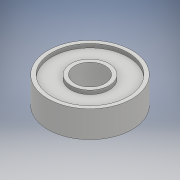
# Autodesk Inventor part: Подшипник
Saved by Autodesk Inventor 2017 (Build 210142000, 142)
## iProperties
Part Number: Подшипник
Material: Типовые
Document SubType Name: Modeling
Designer: Daemon
Density: 1 g/cm^3
Appearance: По умолчанию
Author: Daemon
Autodesk Inventor part; units mm, degrees
ref_plane "YZ Plane" through (0, 0, 0) normal (1, 0, 0) x (0, 1, 0)
ref_plane "XZ Plane" through (0, 0, 0) normal (0, 1, 0) x (-1, 0, 0)
ref_plane "XY Plane" through (0, 0, 0) normal (0, 0, 1) x (1, 0, 0)
sketch "Эскиз1" plane through (0, 0, 0) normal (0, 0, 1) x (1, 0, 0)
  circle A0 centre (0, 0) radius 4
  circle A1 centre (0, 0) radius 11
  dimension "d0" = 8
  dimension "d1" = 22
  constraints: 2 centre point, 2 coincident
  measures "d0" diameter of A0
  measures "d1" diameter of A1
extrude "Выдавливание1" add sketch "Эскиз1" along normal blind 7
sketch "Эскиз3" plane through (0, 0, 7) normal (0, 0, 1) x (1, 0, 0)
  circle A0 centre (0, 0) radius 4 projected
  circle A1 centre (0, 0) radius 4
  circle A2 centre (0, 0) radius 5
  circle A3 centre (0, 0) radius 10
  circle A4 centre (0, 0) radius 11
  dimension "d8" = 10
  dimension "d9" = 20
  dimension "d10" = 22
  dimension "d11" = 8
  constraints: 4 centre point, 4 coincident
  measures "d8" diameter of A2
  measures "d9" diameter of A3
  measures "d10" diameter of A4
  measures "d11" diameter of A1
extrude "Выдавливание3" cut sketch "Эскиз3" against normal blind 1 contours A3
sketch "Эскиз4" plane through (0, 0, 0) normal (0, 0, -1) x (-1, 0, 0)
  circle A0 centre (0, 0) radius 4
  circle A1 centre (0, 0) radius 5
  circle A2 centre (0, 0) radius 11
  circle A3 centre (0, 0) radius 10
  dimension "d14" = 20
  dimension "d15" = 8
  dimension "d16" = 10
  dimension "d17" = 22
  constraints: 4 centre point, 4 coincident
  measures "d14" diameter of A3
  measures "d15" diameter of A0
  measures "d16" diameter of A1
  measures "d17" diameter of A2
extrude "Выдавливание4" cut sketch "Эскиз4" against normal blind 1 contours A3
